Autodesk Fusion 360 part; units mm, degrees
(part 3 of 9)
sketch "Sketch5" plane through (0, 5.1, 0) normal (0, 1, 0) x (-1, 0, 0)
  line L0 (-250.175, 15.525) -> (-250.175, 3.525)
  arc A0 (-251.175, 2.525) -> (-250.175, 3.525) centre (-251.175, 3.525) ccw
  line L1 (-251.175, 2.525) -> (-263.175, 2.525)
  arc A1 (-264.175, 3.525) -> (-263.175, 2.525) centre (-263.175, 3.525) ccw
  line L2 (-264.175, 3.525) -> (-264.175, 15.525)
  arc A2 (-263.175, 16.525) -> (-264.175, 15.525) centre (-263.175, 15.525) ccw
  line L3 (-263.175, 16.525) -> (-251.175, 16.525)
  arc A3 (-250.175, 15.525) -> (-251.175, 16.525) centre (-251.175, 15.525) ccw
  line L4 (-216.8375, 53.625) -> (-216.8375, 41.625)
  arc A4 (-217.8375, 40.625) -> (-216.8375, 41.625) centre (-217.8375, 41.625) ccw
  line L5 (-217.8375, 40.625) -> (-229.8375, 40.625)
  arc A5 (-230.8375, 41.625) -> (-229.8375, 40.625) centre (-229.8375, 41.625) ccw
  line L6 (-230.8375, 41.625) -> (-230.8375, 53.625)
  arc A6 (-229.8375, 54.625) -> (-230.8375, 53.625) centre (-229.8375, 53.625) ccw
  line L7 (-229.8375, 54.625) -> (-217.8375, 54.625)
  arc A7 (-216.8375, 53.625) -> (-217.8375, 54.625) centre (-217.8375, 53.625) ccw
  line L8 (-188.2625, 34.575) -> (-188.2625, 22.575)
  arc A8 (-189.2625, 21.575) -> (-188.2625, 22.575) centre (-189.2625, 22.575) ccw
  line L9 (-189.2625, 21.575) -> (-201.2625, 21.575)
  arc A9 (-202.2625, 22.575) -> (-201.2625, 21.575) centre (-201.2625, 22.575) ccw
  line L10 (-202.2625, 22.575) -> (-202.2625, 34.575)
  arc A10 (-201.2625, 35.575) -> (-202.2625, 34.575) centre (-201.2625, 34.575) ccw
  line L11 (-201.2625, 35.575) -> (-189.2625, 35.575)
  arc A11 (-188.2625, 34.575) -> (-189.2625, 35.575) centre (-189.2625, 34.575) ccw
  line L12 (-178.7375, 53.625) -> (-178.7375, 41.625)
  arc A12 (-179.7375, 40.625) -> (-178.7375, 41.625) centre (-179.7375, 41.625) ccw
  line L13 (-179.7375, 40.625) -> (-191.7375, 40.625)
  arc A13 (-192.7375, 41.625) -> (-191.7375, 40.625) centre (-191.7375, 41.625) ccw
  line L14 (-192.7375, 41.625) -> (-192.7375, 53.625)
  arc A14 (-191.7375, 54.625) -> (-192.7375, 53.625) centre (-191.7375, 53.625) ccw
  line L15 (-191.7375, 54.625) -> (-179.7375, 54.625)
  arc A15 (-178.7375, 53.625) -> (-179.7375, 54.625) centre (-179.7375, 53.625) ccw
  line L16 (-140.6375, 53.625) -> (-140.6375, 41.625)
  arc A16 (-141.6375, 40.625) -> (-140.6375, 41.625) centre (-141.6375, 41.625) ccw
  line L17 (-141.6375, 40.625) -> (-153.6375, 40.625)
  arc A17 (-154.6375, 41.625) -> (-153.6375, 40.625) centre (-153.6375, 41.625) ccw
  line L18 (-154.6375, 41.625) -> (-154.6375, 53.625)
  arc A18 (-153.6375, 54.625) -> (-154.6375, 53.625) centre (-153.6375, 53.625) ccw
  line L19 (-153.6375, 54.625) -> (-141.6375, 54.625)
  arc A19 (-140.6375, 53.625) -> (-141.6375, 54.625) centre (-141.6375, 53.625) ccw
  line L20 (-131.1125, 34.575) -> (-131.1125, 22.575)
  arc A20 (-132.1125, 21.575) -> (-131.1125, 22.575) centre (-132.1125, 22.575) ccw
  line L21 (-132.1125, 21.575) -> (-144.1125, 21.575)
  arc A21 (-145.1125, 22.575) -> (-144.1125, 21.575) centre (-144.1125, 22.575) ccw
  line L22 (-145.1125, 22.575) -> (-145.1125, 34.575)
  arc A22 (-144.1125, 35.575) -> (-145.1125, 34.575) centre (-144.1125, 34.575) ccw
  line L23 (-144.1125, 35.575) -> (-132.1125, 35.575)
  arc A23 (-131.1125, 34.575) -> (-132.1125, 35.575) centre (-132.1125, 34.575) ccw
  line L24 (-107.3, 15.525) -> (-107.3, 3.525)
  arc A24 (-108.3, 2.525) -> (-107.3, 3.525) centre (-108.3, 3.525) ccw
  line L25 (-108.3, 2.525) -> (-120.3, 2.525)
  arc A25 (-121.3, 3.525) -> (-120.3, 2.525) centre (-120.3, 3.525) ccw
  line L26 (-121.3, 3.525) -> (-121.3, 15.525)
  arc A26 (-120.3, 16.525) -> (-121.3, 15.525) centre (-120.3, 15.525) ccw
  line L27 (-120.3, 16.525) -> (-108.3, 16.525)
  arc A27 (-107.3, 15.525) -> (-108.3, 16.525) centre (-108.3, 15.525) ccw
  line L28 (-122.2563, 73.675) -> (-92.0563, 73.675)
  arc A28 (-91.0563, 72.675) -> (-92.0563, 73.675) centre (-92.0563, 72.675) ccw
  line L29 (-91.0563, 72.675) -> (-91.0563, 60.675)
  arc A29 (-92.0563, 59.675) -> (-91.0563, 60.675) centre (-92.0563, 60.675) ccw
  line L30 (-92.0563, 59.675) -> (-122.2563, 59.675)
  arc A30 (-123.2563, 60.675) -> (-122.2563, 59.675) centre (-122.2563, 60.675) ccw
  line L31 (-123.2563, 60.675) -> (-123.2563, 72.675)
  arc A31 (-122.2563, 73.675) -> (-123.2563, 72.675) centre (-122.2563, 72.675) ccw
  line L32 (-69.2, 15.525) -> (-69.2, 3.525)
  arc A32 (-70.2, 2.525) -> (-69.2, 3.525) centre (-70.2, 3.525) ccw
  line L33 (-70.2, 2.525) -> (-82.2, 2.525)
  arc A33 (-83.2, 3.525) -> (-82.2, 2.525) centre (-82.2, 3.525) ccw
  line L34 (-83.2, 3.525) -> (-83.2, 15.525)
  arc A34 (-82.2, 16.525) -> (-83.2, 15.525) centre (-82.2, 15.525) ccw
  line L35 (-82.2, 16.525) -> (-70.2, 16.525)
  arc A35 (-69.2, 15.525) -> (-70.2, 16.525) centre (-70.2, 15.525) ccw
  line L36 (-45.3875, 53.625) -> (-45.3875, 41.625)
  arc A36 (-46.3875, 40.625) -> (-45.3875, 41.625) centre (-46.3875, 41.625) ccw
  line L37 (-46.3875, 40.625) -> (-58.3875, 40.625)
  arc A37 (-59.3875, 41.625) -> (-58.3875, 40.625) centre (-58.3875, 41.625) ccw
  line L38 (-59.3875, 41.625) -> (-59.3875, 53.625)
  arc A38 (-58.3875, 54.625) -> (-59.3875, 53.625) centre (-58.3875, 53.625) ccw
  line L39 (-58.3875, 54.625) -> (-46.3875, 54.625)
  arc A39 (-45.3875, 53.625) -> (-46.3875, 54.625) centre (-46.3875, 53.625) ccw
  line L40 (-9.6688, 34.575) -> (-9.6687, 22.575)
  arc A40 (-10.6687, 21.575) -> (-9.6687, 22.575) centre (-10.6688, 22.575) ccw
  line L41 (-10.6687, 21.575) -> (-22.6688, 21.575)
  arc A41 (-23.6688, 22.575) -> (-22.6688, 21.575) centre (-22.6687, 22.575) ccw
  line L42 (-23.6688, 22.575) -> (-23.6687, 34.575)
  arc A42 (-22.6687, 35.575) -> (-23.6687, 34.575) centre (-22.6687, 34.575) ccw
  line L43 (-22.6688, 35.575) -> (-10.6688, 35.575)
  arc A43 (-9.6688, 34.575) -> (-10.6687, 35.575) centre (-10.6688, 34.575) ccw
  line L44 (-44.1, 16.525) -> (-32.1, 16.525)
  arc A44 (-31.1, 15.525) -> (-32.1, 16.525) centre (-32.1, 15.525) ccw
  line L45 (-31.1, 15.525) -> (-31.1, 3.525)
  arc A45 (-32.1, 2.525) -> (-31.1, 3.525) centre (-32.1, 3.525) ccw
  line L46 (-32.1, 2.525) -> (-44.1, 2.525)
  arc A46 (-45.1, 3.525) -> (-44.1, 2.525) centre (-44.1, 3.525) ccw
  line L47 (-45.1, 3.525) -> (-45.1, 15.525)
  arc A47 (-44.1, 16.525) -> (-45.1, 15.525) centre (-44.1, 15.525) ccw
  line L48 (-40.625, 72.675) -> (-40.625, 60.675)
  arc A48 (-41.625, 59.675) -> (-40.625, 60.675) centre (-41.625, 60.675) ccw
  line L49 (-41.625, 59.675) -> (-53.625, 59.675)
  arc A49 (-54.625, 60.675) -> (-53.625, 59.675) centre (-53.625, 60.675) ccw
  line L50 (-54.625, 60.675) -> (-54.625, 72.675)
  arc A50 (-53.625, 73.675) -> (-54.625, 72.675) centre (-53.625, 72.675) ccw
  line L51 (-53.625, 73.675) -> (-41.625, 73.675)
  arc A51 (-40.625, 72.675) -> (-41.625, 73.675) centre (-41.625, 72.675) ccw
  line L52 (-54.9125, 34.575) -> (-54.9125, 22.575)
  arc A52 (-55.9125, 21.575) -> (-54.9125, 22.575) centre (-55.9125, 22.575) ccw
  line L53 (-55.9125, 21.575) -> (-67.9125, 21.575)
  arc A53 (-68.9125, 22.575) -> (-67.9125, 21.575) centre (-67.9125, 22.575) ccw
  line L54 (-68.9125, 22.575) -> (-68.9125, 34.575)
  arc A54 (-67.9125, 35.575) -> (-68.9125, 34.575) centre (-67.9125, 34.575) ccw
  line L55 (-67.9125, 35.575) -> (-55.9125, 35.575)
  arc A55 (-54.9125, 34.575) -> (-55.9125, 35.575) centre (-55.9125, 34.575) ccw
  line L56 (-66.8188, 72.675) -> (-66.8188, 60.675)
  arc A56 (-67.8188, 59.675) -> (-66.8188, 60.675) centre (-67.8188, 60.675) ccw
  line L57 (-67.8188, 59.675) -> (-79.8188, 59.675)
  arc A57 (-80.8188, 60.675) -> (-79.8188, 59.675) centre (-79.8188, 60.675) ccw
  line L58 (-80.8187, 60.675) -> (-80.8187, 72.675)
  arc A58 (-79.8188, 73.675) -> (-80.8188, 72.675) centre (-79.8188, 72.675) ccw
  line L59 (-79.8188, 73.675) -> (-67.8188, 73.675)
  arc A59 (-66.8188, 72.675) -> (-67.8188, 73.675) centre (-67.8188, 72.675) ccw
  line L60 (-88.25, 15.525) -> (-88.25, 3.525)
  arc A60 (-89.25, 2.525) -> (-88.25, 3.525) centre (-89.25, 3.525) ccw
  line L61 (-89.25, 2.525) -> (-101.25, 2.525)
  arc A61 (-102.25, 3.525) -> (-101.25, 2.525) centre (-101.25, 3.525) ccw
  line L62 (-102.25, 3.525) -> (-102.25, 15.525)
  arc A62 (-101.25, 16.525) -> (-102.25, 15.525) centre (-101.25, 15.525) ccw
  line L63 (-101.25, 16.525) -> (-89.25, 16.525)
  arc A63 (-88.25, 15.525) -> (-89.25, 16.525) centre (-89.25, 15.525) ccw
  line L64 (-121.5875, 53.625) -> (-121.5875, 41.625)
  arc A64 (-122.5875, 40.625) -> (-121.5875, 41.625) centre (-122.5875, 41.625) ccw
  line L65 (-122.5875, 40.625) -> (-134.5875, 40.625)
  arc A65 (-135.5875, 41.625) -> (-134.5875, 40.625) centre (-134.5875, 41.625) ccw
  line L66 (-135.5875, 41.625) -> (-135.5875, 53.625)
  arc A66 (-134.5875, 54.625) -> (-135.5875, 53.625) centre (-134.5875, 53.625) ccw
  line L67 (-134.5875, 54.625) -> (-122.5875, 54.625)
  arc A67 (-121.5875, 53.625) -> (-122.5875, 54.625) centre (-122.5875, 53.625) ccw
  line L68 (-150.1625, 34.575) -> (-150.1625, 22.575)
  arc A68 (-151.1625, 21.575) -> (-150.1625, 22.575) centre (-151.1625, 22.575) ccw
  line L69 (-151.1625, 21.575) -> (-163.1625, 21.575)
  arc A69 (-164.1625, 22.575) -> (-163.1625, 21.575) centre (-163.1625, 22.575) ccw
  line L70 (-164.1625, 22.575) -> (-164.1625, 34.575)
  arc A70 (-163.1625, 35.575) -> (-164.1625, 34.575) centre (-163.1625, 34.575) ccw
  line L71 (-163.1625, 35.575) -> (-151.1625, 35.575)
  arc A71 (-150.1625, 34.575) -> (-151.1625, 35.575) centre (-151.1625, 34.575) ccw
  line L72 (-171.5938, 72.675) -> (-171.5937, 60.675)
  arc A72 (-172.5937, 59.675) -> (-171.5937, 60.675) centre (-172.5937, 60.675) ccw
  line L73 (-172.5938, 59.675) -> (-184.5938, 59.675)
  arc A73 (-185.5938, 60.675) -> (-184.5938, 59.675) centre (-184.5938, 60.675) ccw
  line L74 (-185.5938, 60.675) -> (-185.5937, 72.675)
  arc A74 (-184.5938, 73.675) -> (-185.5937, 72.675) centre (-184.5937, 72.675) ccw
  line L75 (-184.5938, 73.675) -> (-172.5937, 73.675)
  arc A75 (-171.5938, 72.675) -> (-172.5937, 73.675) centre (-172.5937, 72.675) ccw
  line L76 (-183.5, 15.525) -> (-183.5, 3.525)
  arc A76 (-184.5, 2.525) -> (-183.5, 3.525) centre (-184.5, 3.525) ccw
  line L77 (-184.5, 2.525) -> (-196.5, 2.525)
  arc A77 (-197.5, 3.525) -> (-196.5, 2.525) centre (-196.5, 3.525) ccw
  line L78 (-197.5, 3.525) -> (-197.5, 15.525)
  arc A78 (-196.5, 16.525) -> (-197.5, 15.525) centre (-196.5, 15.525) ccw
  line L79 (-196.5, 16.525) -> (-184.5, 16.525)
  arc A79 (-183.5, 15.525) -> (-184.5, 16.525) centre (-184.5, 15.525) ccw
  line L80 (-223.9813, 72.675) -> (-223.9813, 60.675)
  arc A80 (-224.9813, 59.675) -> (-223.9812, 60.675) centre (-224.9812, 60.675) ccw
  line L81 (-224.9813, 59.675) -> (-236.9813, 59.675)
  arc A81 (-237.9813, 60.675) -> (-236.9813, 59.675) centre (-236.9813, 60.675) ccw
  line L82 (-237.9813, 60.675) -> (-237.9812, 72.675)
  arc A82 (-236.9813, 73.675) -> (-237.9813, 72.675) centre (-236.9813, 72.675) ccw
  line L83 (-236.9813, 73.675) -> (-224.9813, 73.675)
  arc A83 (-223.9813, 72.675) -> (-224.9813, 73.675) centre (-224.9812, 72.675) ccw
  line L84 (-226.3625, 15.525) -> (-226.3625, 3.525)
  arc A84 (-227.3625, 2.525) -> (-226.3625, 3.525) centre (-227.3625, 3.525) ccw
  line L85 (-227.3625, 2.525) -> (-239.3625, 2.525)
  arc A85 (-240.3625, 3.525) -> (-239.3625, 2.525) centre (-239.3625, 3.525) ccw
  line L86 (-240.3625, 3.525) -> (-240.3625, 15.525)
  arc A86 (-239.3625, 16.525) -> (-240.3625, 15.525) centre (-239.3625, 15.525) ccw
  line L87 (-239.3625, 16.525) -> (-227.3625, 16.525)
  arc A87 (-226.3625, 15.525) -> (-227.3625, 16.525) centre (-227.3625, 15.525) ccw
  line L88 (-260.3688, 35.575) -> (-230.1688, 35.575)
  arc A88 (-229.1688, 34.575) -> (-230.1688, 35.575) centre (-230.1688, 34.575) ccw
  line L89 (-229.1688, 34.575) -> (-229.1688, 22.575)
  arc A89 (-230.1688, 21.575) -> (-229.1688, 22.575) centre (-230.1688, 22.575) ccw
  line L90 (-230.1688, 21.575) -> (-260.3688, 21.575)
  arc A90 (-261.3688, 22.575) -> (-260.3688, 21.575) centre (-260.3688, 22.575) ccw
  line L91 (-261.3688, 22.575) -> (-261.3688, 34.575)
  arc A91 (-260.3688, 35.575) -> (-261.3688, 34.575) centre (-260.3687, 34.575) ccw
  line L92 (-207.3125, 34.575) -> (-207.3125, 22.575)
  arc A92 (-208.3125, 21.575) -> (-207.3125, 22.575) centre (-208.3125, 22.575) ccw
  line L93 (-208.3125, 21.575) -> (-220.3125, 21.575)
  arc A93 (-221.3125, 22.575) -> (-220.3125, 21.575) centre (-220.3125, 22.575) ccw
  line L94 (-221.3125, 22.575) -> (-221.3125, 34.575)
  arc A94 (-220.3125, 35.575) -> (-221.3125, 34.575) centre (-220.3125, 34.575) ccw
  line L95 (-220.3125, 35.575) -> (-208.3125, 35.575)
  arc A95 (-207.3125, 34.575) -> (-208.3125, 35.575) centre (-208.3125, 34.575) ccw
  line L96 (-197.7875, 53.625) -> (-197.7875, 41.625)
  arc A96 (-198.7875, 40.625) -> (-197.7875, 41.625) centre (-198.7875, 41.625) ccw
  line L97 (-198.7875, 40.625) -> (-210.7875, 40.625)
  arc A97 (-211.7875, 41.625) -> (-210.7875, 40.625) centre (-210.7875, 41.625) ccw
  line L98 (-211.7875, 41.625) -> (-211.7875, 53.625)
  arc A98 (-210.7875, 54.625) -> (-211.7875, 53.625) centre (-210.7875, 53.625) ccw
  line L99 (-210.7875, 54.625) -> (-198.7875, 54.625)
  arc A99 (-197.7875, 53.625) -> (-198.7875, 54.625) centre (-198.7875, 53.625) ccw
  line L100 (-169.2125, 34.575) -> (-169.2125, 22.575)
  arc A100 (-170.2125, 21.575) -> (-169.2125, 22.575) centre (-170.2125, 22.575) ccw
  line L101 (-170.2125, 21.575) -> (-182.2125, 21.575)
  arc A101 (-183.2125, 22.575) -> (-182.2125, 21.575) centre (-182.2125, 22.575) ccw
  line L102 (-183.2125, 22.575) -> (-183.2125, 34.575)
  arc A102 (-182.2125, 35.575) -> (-183.2125, 34.575) centre (-182.2125, 34.575) ccw
  line L103 (-182.2125, 35.575) -> (-170.2125, 35.575)
  arc A103 (-169.2125, 34.575) -> (-170.2125, 35.575) centre (-170.2125, 34.575) ccw
  line L104 (-132.5375, 59.675) -> (-162.7375, 59.675)
  arc A104 (-163.7375, 60.675) -> (-162.7375, 59.675) centre (-162.7375, 60.675) ccw
  line L105 (-163.7375, 60.675) -> (-163.7375, 72.675)
  arc A105 (-162.7375, 73.675) -> (-163.7375, 72.675) centre (-162.7375, 72.675) ccw
  line L106 (-162.7375, 73.675) -> (-132.5375, 73.675)
  arc A106 (-131.5375, 72.675) -> (-132.5375, 73.675) centre (-132.5375, 72.675) ccw
  line L107 (-131.5375, 72.675) -> (-131.5375, 60.675)
  arc A107 (-132.5375, 59.675) -> (-131.5375, 60.675) centre (-132.5375, 60.675) ccw
  line L108 (-126.35, 15.525) -> (-126.35, 3.525)
  arc A108 (-127.35, 2.525) -> (-126.35, 3.525) centre (-127.35, 3.525) ccw
  line L109 (-127.35, 2.525) -> (-139.35, 2.525)
  arc A109 (-140.35, 3.525) -> (-139.35, 2.525) centre (-139.35, 3.525) ccw
  line L110 (-140.35, 3.525) -> (-140.35, 15.525)
  arc A110 (-139.35, 16.525) -> (-140.35, 15.525) centre (-139.35, 15.525) ccw
  line L111 (-139.35, 16.525) -> (-127.35, 16.525)
  arc A111 (-126.35, 15.525) -> (-127.35, 16.525) centre (-127.35, 15.525) ccw
  line L112 (-112.0625, 34.575) -> (-112.0625, 22.575)
  arc A112 (-113.0625, 21.575) -> (-112.0625, 22.575) centre (-113.0625, 22.575) ccw
  line L113 (-113.0625, 21.575) -> (-125.0625, 21.575)
  arc A113 (-126.0625, 22.575) -> (-125.0625, 21.575) centre (-125.0625, 22.575) ccw
  line L114 (-126.0625, 22.575) -> (-126.0625, 34.575)
  arc A114 (-125.0625, 35.575) -> (-126.0625, 34.575) centre (-125.0625, 34.575) ccw
  line L115 (-125.0625, 35.575) -> (-113.0625, 35.575)
  arc A115 (-112.0625, 34.575) -> (-113.0625, 35.575) centre (-113.0625, 34.575) ccw
  line L116 (-83.4875, 53.625) -> (-83.4875, 41.625)
  arc A116 (-84.4875, 40.625) -> (-83.4875, 41.625) centre (-84.4875, 41.625) ccw
  line L117 (-84.4875, 40.625) -> (-96.4875, 40.625)
  arc A117 (-97.4875, 41.625) -> (-96.4875, 40.625) centre (-96.4875, 41.625) ccw
  line L118 (-97.4875, 41.625) -> (-97.4875, 53.625)
  arc A118 (-96.4875, 54.625) -> (-97.4875, 53.625) centre (-96.4875, 53.625) ccw
  line L119 (-96.4875, 54.625) -> (-84.4875, 54.625)
  arc A119 (-83.4875, 53.625) -> (-84.4875, 54.625) centre (-84.4875, 53.625) ccw
  line L120 (-73.9625, 34.575) -> (-73.9625, 22.575)
  arc A120 (-74.9625, 21.575) -> (-73.9625, 22.575) centre (-74.9625, 22.575) ccw
  line L121 (-74.9625, 21.575) -> (-86.9625, 21.575)
  arc A121 (-87.9625, 22.575) -> (-86.9625, 21.575) centre (-86.9625, 22.575) ccw
  line L122 (-87.9625, 22.575) -> (-87.9625, 34.575)
  arc A122 (-86.9625, 35.575) -> (-87.9625, 34.575) centre (-86.9625, 34.575) ccw
  line L123 (-86.9625, 35.575) -> (-74.9625, 35.575)
  arc A123 (-73.9625, 34.575) -> (-74.9625, 35.575) centre (-74.9625, 34.575) ccw
  line L124 (-35.8625, 34.575) -> (-35.8625, 22.575)
  arc A124 (-36.8625, 21.575) -> (-35.8625, 22.575) centre (-36.8625, 22.575) ccw
  line L125 (-36.8625, 21.575) -> (-48.8625, 21.575)
  arc A125 (-49.8625, 22.575) -> (-48.8625, 21.575) centre (-48.8625, 22.575) ccw
  line L126 (-49.8625, 22.575) -> (-49.8625, 34.575)
  arc A126 (-48.8625, 35.575) -> (-49.8625, 34.575) centre (-48.8625, 34.575) ccw
  line L127 (-48.8625, 35.575) -> (-36.8625, 35.575)
  arc A127 (-35.8625, 34.575) -> (-36.8625, 35.575) centre (-36.8625, 34.575) ccw
  line L128 (-6.3312, 40.625) -> (-36.5313, 40.625)
  arc A128 (-37.5313, 41.625) -> (-36.5313, 40.625) centre (-36.5313, 41.625) ccw
  line L129 (-37.5312, 41.625) -> (-37.5312, 53.625)
  arc A129 (-36.5313, 54.625) -> (-37.5313, 53.625) centre (-36.5313, 53.625) ccw
  line L130 (-36.5313, 54.625) -> (-6.3313, 54.625)
  arc A130 (-5.3313, 53.625) -> (-6.3313, 54.625) centre (-6.3312, 53.625) ccw
  line L131 (-5.3313, 53.625) -> (-5.3312, 41.625)
  arc A131 (-6.3312, 40.625) -> (-5.3312, 41.625) centre (-6.3312, 41.625) ccw
  line L132 (-7.2875, 15.525) -> (-7.2875, 3.525)
  arc A132 (-8.2875, 2.525) -> (-7.2875, 3.525) centre (-8.2875, 3.525) ccw
  line L133 (-8.2875, 2.525) -> (-20.2875, 2.525)
  arc A133 (-21.2875, 3.525) -> (-20.2875, 2.525) centre (-20.2875, 3.525) ccw
  line L134 (-21.2875, 3.525) -> (-21.2875, 15.525)
  arc A134 (-20.2875, 16.525) -> (-21.2875, 15.525) centre (-20.2875, 15.525) ccw
  line L135 (-20.2875, 16.525) -> (-8.2875, 16.525)
  arc A135 (-7.2875, 15.525) -> (-8.2875, 16.525) centre (-8.2875, 15.525) ccw
  line L136 (-14.4313, 72.675) -> (-14.4313, 60.675)
  arc A136 (-15.4313, 59.675) -> (-14.4313, 60.675) centre (-15.4312, 60.675) ccw
  line L137 (-15.4313, 59.675) -> (-27.4313, 59.675)
  arc A137 (-28.4313, 60.675) -> (-27.4313, 59.675) centre (-27.4313, 60.675) ccw
  line L138 (-28.4313, 60.675) -> (-28.4312, 72.675)
  arc A138 (-27.4313, 73.675) -> (-28.4312, 72.675) centre (-27.4312, 72.675) ccw
  line L139 (-27.4313, 73.675) -> (-15.4313, 73.675)
  arc A139 (-14.4313, 72.675) -> (-15.4313, 73.675) centre (-15.4313, 72.675) ccw
  line L140 (-50.15, 15.525) -> (-50.15, 3.525)
  arc A140 (-51.15, 2.525) -> (-50.15, 3.525) centre (-51.15, 3.525) ccw
  line L141 (-51.15, 2.525) -> (-63.15, 2.525)
  arc A141 (-64.15, 3.525) -> (-63.15, 2.525) centre (-63.15, 3.525) ccw
  line L142 (-64.15, 3.525) -> (-64.15, 15.525)
  arc A142 (-63.15, 16.525) -> (-64.15, 15.525) centre (-63.15, 15.525) ccw
  line L143 (-63.15, 16.525) -> (-51.15, 16.525)
  arc A143 (-50.15, 15.525) -> (-51.15, 16.525) centre (-51.15, 15.525) ccw
  line L144 (-64.4375, 53.625) -> (-64.4375, 41.625)
  arc A144 (-65.4375, 40.625) -> (-64.4375, 41.625) centre (-65.4375, 41.625) ccw
  line L145 (-65.4375, 40.625) -> (-77.4375, 40.625)
  arc A145 (-78.4375, 41.625) -> (-77.4375, 40.625) centre (-77.4375, 41.625) ccw
  line L146 (-78.4375, 41.625) -> (-78.4375, 53.625)
  arc A146 (-77.4375, 54.625) -> (-78.4375, 53.625) centre (-77.4375, 53.625) ccw
  line L147 (-77.4375, 54.625) -> (-65.4375, 54.625)
  arc A147 (-64.4375, 53.625) -> (-65.4375, 54.625) centre (-65.4375, 53.625) ccw
  line L148 (-93.0125, 34.575) -> (-93.0125, 22.575)
  arc A148 (-94.0125, 21.575) -> (-93.0125, 22.575) centre (-94.0125, 22.575) ccw
  line L149 (-94.0125, 21.575) -> (-106.0125, 21.575)
  arc A149 (-107.0125, 22.575) -> (-106.0125, 21.575) centre (-106.0125, 22.575) ccw
  line L150 (-107.0125, 22.575) -> (-107.0125, 34.575)
  arc A150 (-106.0125, 35.575) -> (-107.0125, 34.575) centre (-106.0125, 34.575) ccw
  line L151 (-106.0125, 35.575) -> (-94.0125, 35.575)
  arc A151 (-93.0125, 34.575) -> (-94.0125, 35.575) centre (-94.0125, 34.575) ccw
  line L152 (-102.5375, 53.625) -> (-102.5375, 41.625)
  arc A152 (-103.5375, 40.625) -> (-102.5375, 41.625) centre (-103.5375, 41.625) ccw
  line L153 (-103.5375, 40.625) -> (-115.5375, 40.625)
  arc A153 (-116.5375, 41.625) -> (-115.5375, 40.625) centre (-115.5375, 41.625) ccw
  line L154 (-116.5375, 41.625) -> (-116.5375, 53.625)
  arc A154 (-115.5375, 54.625) -> (-116.5375, 53.625) centre (-115.5375, 53.625) ccw
  line L155 (-115.5375, 54.625) -> (-103.5375, 54.625)
  arc A155 (-102.5375, 53.625) -> (-103.5375, 54.625) centre (-103.5375, 53.625) ccw
  line L156 (-145.4, 15.525) -> (-145.4, 3.525)
  arc A156 (-146.4, 2.525) -> (-145.4, 3.525) centre (-146.4, 3.525) ccw
  line L157 (-146.4, 2.525) -> (-158.4, 2.525)
  arc A157 (-159.4, 3.525) -> (-158.4, 2.525) centre (-158.4, 3.525) ccw
  line L158 (-159.4, 3.525) -> (-159.4, 15.525)
  arc A158 (-158.4, 16.525) -> (-159.4, 15.525) centre (-158.4, 15.525) ccw
  line L159 (-158.4, 16.525) -> (-146.4, 16.525)
  arc A159 (-145.4, 15.525) -> (-146.4, 16.525) centre (-146.4, 15.525) ccw
  line L160 (-159.6875, 53.625) -> (-159.6875, 41.625)
  arc A160 (-160.6875, 40.625) -> (-159.6875, 41.625) centre (-160.6875, 41.625) ccw
  line L161 (-160.6875, 40.625) -> (-172.6875, 40.625)
  arc A161 (-173.6875, 41.625) -> (-172.6875, 40.625) centre (-172.6875, 41.625) ccw
  line L162 (-173.6875, 41.625) -> (-173.6875, 53.625)
  arc A162 (-172.6875, 54.625) -> (-173.6875, 53.625) centre (-172.6875, 53.625) ccw
  line L163 (-172.6875, 54.625) -> (-160.6875, 54.625)
  arc A163 (-159.6875, 53.625) -> (-160.6875, 54.625) centre (-160.6875, 53.625) ccw
  line L164 (-164.45, 15.525) -> (-164.45, 3.525)
  arc A164 (-165.45, 2.525) -> (-164.45, 3.525) centre (-165.45, 3.525) ccw
  line L165 (-165.45, 2.525) -> (-177.45, 2.525)
  arc A165 (-178.45, 3.525) -> (-177.45, 2.525) centre (-177.45, 3.525) ccw
  line L166 (-178.45, 3.525) -> (-178.45, 15.525)
  arc A166 (-177.45, 16.525) -> (-178.45, 15.525) centre (-177.45, 15.525) ccw
  line L167 (-177.45, 16.525) -> (-165.45, 16.525)
  arc A167 (-164.45, 15.525) -> (-165.45, 16.525) centre (-165.45, 15.525) ccw
  line L168 (-197.7875, 72.675) -> (-197.7875, 60.675)
  arc A168 (-198.7875, 59.675) -> (-197.7875, 60.675) centre (-198.7875, 60.675) ccw
  line L169 (-198.7875, 59.675) -> (-210.7875, 59.675)
  arc A169 (-211.7875, 60.675) -> (-210.7875, 59.675) centre (-210.7875, 60.675) ccw
  line L170 (-211.7875, 60.675) -> (-211.7875, 72.675)
  arc A170 (-210.7875, 73.675) -> (-211.7875, 72.675) centre (-210.7875, 72.675) ccw
  line L171 (-210.7875, 73.675) -> (-198.7875, 73.675)
  arc A171 (-197.7875, 72.675) -> (-198.7875, 73.675) centre (-198.7875, 72.675) ccw
  line L172 (-202.55, 15.525) -> (-202.55, 3.525)
  arc A172 (-203.55, 2.525) -> (-202.55, 3.525) centre (-203.55, 3.525) ccw
  line L173 (-203.55, 2.525) -> (-215.55, 2.525)
  arc A173 (-216.55, 3.525) -> (-215.55, 2.525) centre (-215.55, 3.525) ccw
  line L174 (-216.55, 3.525) -> (-216.55, 15.525)
  arc A174 (-215.55, 16.525) -> (-216.55, 15.525) centre (-215.55, 15.525) ccw
  line L175 (-215.55, 16.525) -> (-203.55, 16.525)
  arc A175 (-202.55, 15.525) -> (-203.55, 16.525) centre (-203.55, 15.525) ccw
  line L176 (-243.0312, 53.625) -> (-243.0312, 41.625)
  arc A176 (-244.0312, 40.625) -> (-243.0313, 41.625) centre (-244.0313, 41.625) ccw
  line L177 (-244.0312, 40.625) -> (-256.0312, 40.625)
  arc A177 (-257.0312, 41.625) -> (-256.0312, 40.625) centre (-256.0312, 41.625) ccw
  line L178 (-257.0312, 41.625) -> (-257.0312, 53.625)
  arc A178 (-256.0312, 54.625) -> (-257.0312, 53.625) centre (-256.0312, 53.625) ccw
  line L179 (-256.0312, 54.625) -> (-244.0312, 54.625)
  arc A179 (-243.0313, 53.625) -> (-244.0312, 54.625) centre (-244.0312, 53.625) ccw
  arc A180 (-263.7, 57.15) -> (-266.7, 54.15) centre (-263.7, 54.15) ccw
  line L180 (-266.7, 54.15) -> (-266.7, 3)
  arc A181 (-266.7, 3) -> (-263.7, 0) centre (-263.7, 3) ccw
  line L181 (-263.7, 0) -> (-3, 0)
  arc A182 (-3, 0) -> (0, 3) centre (-3, 3) ccw
  line L182 (0, 3) -> (0, 54.15)
  arc A183 (0, 54.15) -> (-3, 57.15) centre (-3, 54.15) ccw
  line L183 (-3, 57.15) -> (-8.525, 57.15)
  arc A184 (-9.525, 58.15) -> (-8.525, 57.15) centre (-8.525, 58.15) ccw
  line L184 (-9.525, 58.15) -> (-9.525, 73.2)
  arc A185 (-9.525, 73.2) -> (-12.525, 76.2) centre (-12.525, 73.2) ccw
  line L185 (-12.525, 76.2) -> (-239.8875, 76.2)
  arc A186 (-239.8875, 76.2) -> (-242.8875, 73.2) centre (-239.8875, 73.2) ccw
  line L186 (-242.8875, 73.2) -> (-242.8875, 58.15)
  arc A187 (-243.8875, 57.15) -> (-242.8875, 58.15) centre (-243.8875, 58.15) ccw
  line L187 (-243.8875, 57.15) -> (-263.7, 57.15)
  circle A188 centre (-47.625, 9.525) radius 2.5
  circle A189 centre (-245.269, 9.525) radius 2.5
  circle A190 centre (-128.588, 37.025) radius 2.5
  circle A191 centre (-32.525, 66.675) radius 2.5
  circle A192 centre (-220.025, 66.675) radius 2.5
  point P0 (-9.525, 9.525)
  dimension "d82" = 9.525
  dimension "d83" = 9.525
  dimension "d84" = 5
  dimension "d85" = 38.1
  dimension "d86" = 5
  dimension "d87" = 235.744
  dimension "d88" = 5
  dimension "d89" = 119.063
  dimension "d90" = 27.5
  dimension "d91" = 5
  dimension "d92" = 5
  dimension "d93" = 57.15
  dimension "d94" = 57.15
  dimension "d95" = 23
  dimension "d96" = 210.5
  measures "d82" distance of L181 P0
  measures "d83" distance of L182 P0
  measures "d84" diameter of A188
  measures "d85" distance of P0 A188.centre
  measures "d86" diameter of A189
  measures "d87" distance of P0 A189.centre
  measures "d88" diameter of A190
  measures "d89" horizontal distance of P0 A190.centre
  measures "d90" vertical distance of P0 A190.centre
  measures "d91" diameter of A191
  measures "d92" diameter of A192
  measures "d93" vertical distance of P0 A191.centre
  measures "d94" vertical distance of P0 A192.centre
  measures "d95" horizontal distance of P0 A191.centre
  measures "d96" horizontal distance of P0 A192.centre
hole "Hole1" at (245.269, 5.1, 9.525) at (220.025, 5.1, 66.675) at (128.588, 5.1, 37.025) at (47.625, 5.1, 9.525) at (32.525, 5.1, 66.675) direction (0, -1, 0) diameter 2.5 depth 5.1 tip angle 118 counterbore diameter 5 counterbore depth 1.5
sketch "Sketch6" plane through (0, 5.1, 0) normal (0, 1, 0) x (-1, 0, 0)
  circle A0 centre (-47.625, 9.525) radius 2.5
  circle A1 centre (-220.025, 66.675) radius 2.5
  circle A2 centre (-245.269, 9.525) radius 2.5
  circle A3 centre (-128.588, 37.025) radius 2.5
  circle A4 centre (-32.525, 66.675) radius 2.5
  line L0 (-250.175, 15.525) -> (-250.175, 3.525)
  arc A5 (-251.175, 2.525) -> (-250.175, 3.525) centre (-251.175, 3.525) ccw
  line L1 (-251.175, 2.525) -> (-263.175, 2.525)
  arc A6 (-264.175, 3.525) -> (-263.175, 2.525) centre (-263.175, 3.525) ccw
  line L2 (-264.175, 3.525) -> (-264.175, 15.525)
  arc A7 (-263.175, 16.525) -> (-264.175, 15.525) centre (-263.175, 15.525) ccw
  line L3 (-263.175, 16.525) -> (-251.175, 16.525)
  arc A8 (-250.175, 15.525) -> (-251.175, 16.525) centre (-251.175, 15.525) ccw
  line L4 (-216.8375, 53.625) -> (-216.8375, 41.625)
  arc A9 (-217.8375, 40.625) -> (-216.8375, 41.625) centre (-217.8375, 41.625) ccw
  line L5 (-217.8375, 40.625) -> (-229.8375, 40.625)
  arc A10 (-230.8375, 41.625) -> (-229.8375, 40.625) centre (-229.8375, 41.625) ccw
  line L6 (-230.8375, 41.625) -> (-230.8375, 53.625)
  arc A11 (-229.8375, 54.625) -> (-230.8375, 53.625) centre (-229.8375, 53.625) ccw
  line L7 (-229.8375, 54.625) -> (-217.8375, 54.625)
  arc A12 (-216.8375, 53.625) -> (-217.8375, 54.625) centre (-217.8375, 53.625) ccw
  line L8 (-188.2625, 34.575) -> (-188.2625, 22.575)
  arc A13 (-189.2625, 21.575) -> (-188.2625, 22.575) centre (-189.2625, 22.575) ccw
  line L9 (-189.2625, 21.575) -> (-201.2625, 21.575)
  arc A14 (-202.2625, 22.575) -> (-201.2625, 21.575) centre (-201.2625, 22.575) ccw
  line L10 (-202.2625, 22.575) -> (-202.2625, 34.575)
  arc A15 (-201.2625, 35.575) -> (-202.2625, 34.575) centre (-201.2625, 34.575) ccw
  line L11 (-201.2625, 35.575) -> (-189.2625, 35.575)
  arc A16 (-188.2625, 34.575) -> (-189.2625, 35.575) centre (-189.2625, 34.575) ccw
  line L12 (-178.7375, 53.625) -> (-178.7375, 41.625)
  arc A17 (-179.7375, 40.625) -> (-178.7375, 41.625) centre (-179.7375, 41.625) ccw
  line L13 (-179.7375, 40.625) -> (-191.7375, 40.625)
  arc A18 (-192.7375, 41.625) -> (-191.7375, 40.625) centre (-191.7375, 41.625) ccw
  line L14 (-192.7375, 41.625) -> (-192.7375, 53.625)
  arc A19 (-191.7375, 54.625) -> (-192.7375, 53.625) centre (-191.7375, 53.625) ccw
  line L15 (-191.7375, 54.625) -> (-179.7375, 54.625)
  arc A20 (-178.7375, 53.625) -> (-179.7375, 54.625) centre (-179.7375, 53.625) ccw
  line L16 (-140.6375, 53.625) -> (-140.6375, 41.625)
  arc A21 (-141.6375, 40.625) -> (-140.6375, 41.625) centre (-141.6375, 41.625) ccw
  line L17 (-141.6375, 40.625) -> (-153.6375, 40.625)
  arc A22 (-154.6375, 41.625) -> (-153.6375, 40.625) centre (-153.6375, 41.625) ccw
  line L18 (-154.6375, 41.625) -> (-154.6375, 53.625)
  arc A23 (-153.6375, 54.625) -> (-154.6375, 53.625) centre (-153.6375, 53.625) ccw
  line L19 (-153.6375, 54.625) -> (-141.6375, 54.625)
  arc A24 (-140.6375, 53.625) -> (-141.6375, 54.625) centre (-141.6375, 53.625) ccw
  line L20 (-131.1125, 34.575) -> (-131.1125, 22.575)
  arc A25 (-132.1125, 21.575) -> (-131.1125, 22.575) centre (-132.1125, 22.575) ccw
  line L21 (-132.1125, 21.575) -> (-144.1125, 21.575)
  arc A26 (-145.1125, 22.575) -> (-144.1125, 21.575) centre (-144.1125, 22.575) ccw
  line L22 (-145.1125, 22.575) -> (-145.1125, 34.575)
  arc A27 (-144.1125, 35.575) -> (-145.1125, 34.575) centre (-144.1125, 34.575) ccw
  line L23 (-144.1125, 35.575) -> (-132.1125, 35.575)
  arc A28 (-131.1125, 34.575) -> (-132.1125, 35.575) centre (-132.1125, 34.575) ccw
  line L24 (-107.3, 15.525) -> (-107.3, 3.525)
  arc A29 (-108.3, 2.525) -> (-107.3, 3.525) centre (-108.3, 3.525) ccw
  line L25 (-108.3, 2.525) -> (-120.3, 2.525)
  arc A30 (-121.3, 3.525) -> (-120.3, 2.525) centre (-120.3, 3.525) ccw
  line L26 (-121.3, 3.525) -> (-121.3, 15.525)
  arc A31 (-120.3, 16.525) -> (-121.3, 15.525) centre (-120.3, 15.525) ccw
  line L27 (-120.3, 16.525) -> (-108.3, 16.525)
  arc A32 (-107.3, 15.525) -> (-108.3, 16.525) centre (-108.3, 15.525) ccw
  line L28 (-122.2563, 73.675) -> (-92.0563, 73.675)
  arc A33 (-91.0563, 72.675) -> (-92.0563, 73.675) centre (-92.0563, 72.675) ccw
  line L29 (-91.0563, 72.675) -> (-91.0563, 60.675)
  arc A34 (-92.0563, 59.675) -> (-91.0563, 60.675) centre (-92.0563, 60.675) ccw
  line L30 (-92.0563, 59.675) -> (-122.2563, 59.675)
  arc A35 (-123.2563, 60.675) -> (-122.2563, 59.675) centre (-122.2563, 60.675) ccw
  line L31 (-123.2563, 60.675) -> (-123.2563, 72.675)
  arc A36 (-122.2563, 73.675) -> (-123.2563, 72.675) centre (-122.2563, 72.675) ccw
  line L32 (-69.2, 15.525) -> (-69.2, 3.525)
  arc A37 (-70.2, 2.525) -> (-69.2, 3.525) centre (-70.2, 3.525) ccw
  line L33 (-70.2, 2.525) -> (-82.2, 2.525)
  arc A38 (-83.2, 3.525) -> (-82.2, 2.525) centre (-82.2, 3.525) ccw
  line L34 (-83.2, 3.525) -> (-83.2, 15.525)
  arc A39 (-82.2, 16.525) -> (-83.2, 15.525) centre (-82.2, 15.525) ccw
  line L35 (-82.2, 16.525) -> (-70.2, 16.525)
  arc A40 (-69.2, 15.525) -> (-70.2, 16.525) centre (-70.2, 15.525) ccw
  line L36 (-45.3875, 53.625) -> (-45.3875, 41.625)
  arc A41 (-46.3875, 40.625) -> (-45.3875, 41.625) centre (-46.3875, 41.625) ccw
  line L37 (-46.3875, 40.625) -> (-58.3875, 40.625)
  arc A42 (-59.3875, 41.625) -> (-58.3875, 40.625) centre (-58.3875, 41.625) ccw
  line L38 (-59.3875, 41.625) -> (-59.3875, 53.625)
  arc A43 (-58.3875, 54.625) -> (-59.3875, 53.625) centre (-58.3875, 53.625) ccw
  line L39 (-58.3875, 54.625) -> (-46.3875, 54.625)
  arc A44 (-45.3875, 53.625) -> (-46.3875, 54.625) centre (-46.3875, 53.625) ccw
  line L40 (-9.6688, 34.575) -> (-9.6687, 22.575)
  arc A45 (-10.6687, 21.575) -> (-9.6687, 22.575) centre (-10.6688, 22.575) ccw
  line L41 (-10.6687, 21.575) -> (-22.6688, 21.575)
  arc A46 (-23.6688, 22.575) -> (-22.6688, 21.575) centre (-22.6687, 22.575) ccw
  line L42 (-23.6688, 22.575) -> (-23.6687, 34.575)
  arc A47 (-22.6687, 35.575) -> (-23.6687, 34.575) centre (-22.6687, 34.575) ccw
  line L43 (-22.6688, 35.575) -> (-10.6688, 35.575)
  arc A48 (-9.6688, 34.575) -> (-10.6687, 35.575) centre (-10.6688, 34.575) ccw
  line L44 (-44.1, 16.525) -> (-32.1, 16.525)
  arc A49 (-31.1, 15.525) -> (-32.1, 16.525) centre (-32.1, 15.525) ccw
  line L45 (-31.1, 15.525) -> (-31.1, 3.525)
  arc A50 (-32.1, 2.525) -> (-31.1, 3.525) centre (-32.1, 3.525) ccw
  line L46 (-32.1, 2.525) -> (-44.1, 2.525)
  arc A51 (-45.1, 3.525) -> (-44.1, 2.525) centre (-44.1, 3.525) ccw
  line L47 (-45.1, 3.525) -> (-45.1, 15.525)
  arc A52 (-44.1, 16.525) -> (-45.1, 15.525) centre (-44.1, 15.525) ccw
  line L48 (-40.625, 72.675) -> (-40.625, 60.675)
  arc A53 (-41.625, 59.675) -> (-40.625, 60.675) centre (-41.625, 60.675) ccw
  line L49 (-41.625, 59.675) -> (-53.625, 59.675)
  arc A54 (-54.625, 60.675) -> (-53.625, 59.675) centre (-53.625, 60.675) ccw
  line L50 (-54.625, 60.675) -> (-54.625, 72.675)
  arc A55 (-53.625, 73.675) -> (-54.625, 72.675) centre (-53.625, 72.675) ccw
  line L51 (-53.625, 73.675) -> (-41.625, 73.675)
  arc A56 (-40.625, 72.675) -> (-41.625, 73.675) centre (-41.625, 72.675) ccw
  line L52 (-54.9125, 34.575) -> (-54.9125, 22.575)
  arc A57 (-55.9125, 21.575) -> (-54.9125, 22.575) centre (-55.9125, 22.575) ccw
  line L53 (-55.9125, 21.575) -> (-67.9125, 21.575)
  arc A58 (-68.9125, 22.575) -> (-67.9125, 21.575) centre (-67.9125, 22.575) ccw
  line L54 (-68.9125, 22.575) -> (-68.9125, 34.575)
  arc A59 (-67.9125, 35.575) -> (-68.9125, 34.575) centre (-67.9125, 34.575) ccw
  line L55 (-67.9125, 35.575) -> (-55.9125, 35.575)
  arc A60 (-54.9125, 34.575) -> (-55.9125, 35.575) centre (-55.9125, 34.575) ccw
  line L56 (-66.8188, 72.675) -> (-66.8188, 60.675)
  arc A61 (-67.8188, 59.675) -> (-66.8188, 60.675) centre (-67.8188, 60.675) ccw
  line L57 (-67.8188, 59.675) -> (-79.8188, 59.675)
  arc A62 (-80.8188, 60.675) -> (-79.8188, 59.675) centre (-79.8188, 60.675) ccw
  line L58 (-80.8187, 60.675) -> (-80.8187, 72.675)
  arc A63 (-79.8188, 73.675) -> (-80.8188, 72.675) centre (-79.8188, 72.675) ccw
  line L59 (-79.8188, 73.675) -> (-67.8188, 73.675)
  arc A64 (-66.8188, 72.675) -> (-67.8188, 73.675) centre (-67.8188, 72.675) ccw
  line L60 (-88.25, 15.525) -> (-88.25, 3.525)
  arc A65 (-89.25, 2.525) -> (-88.25, 3.525) centre (-89.25, 3.525) ccw
  line L61 (-89.25, 2.525) -> (-101.25, 2.525)
  arc A66 (-102.25, 3.525) -> (-101.25, 2.525) centre (-101.25, 3.525) ccw
  line L62 (-102.25, 3.525) -> (-102.25, 15.525)
  arc A67 (-101.25, 16.525) -> (-102.25, 15.525) centre (-101.25, 15.525) ccw
  line L63 (-101.25, 16.525) -> (-89.25, 16.525)
  arc A68 (-88.25, 15.525) -> (-89.25, 16.525) centre (-89.25, 15.525) ccw
  line L64 (-121.5875, 53.625) -> (-121.5875, 41.625)
  arc A69 (-122.5875, 40.625) -> (-121.5875, 41.625) centre (-122.5875, 41.625) ccw
  line L65 (-122.5875, 40.625) -> (-134.5875, 40.625)
  arc A70 (-135.5875, 41.625) -> (-134.5875, 40.625) centre (-134.5875, 41.625) ccw
  line L66 (-135.5875, 41.625) -> (-135.5875, 53.625)
  arc A71 (-134.5875, 54.625) -> (-135.5875, 53.625) centre (-134.5875, 53.625) ccw
  line L67 (-134.5875, 54.625) -> (-122.5875, 54.625)
  arc A72 (-121.5875, 53.625) -> (-122.5875, 54.625) centre (-122.5875, 53.625) ccw
  line L68 (-150.1625, 34.575) -> (-150.1625, 22.575)
  arc A73 (-151.1625, 21.575) -> (-150.1625, 22.575) centre (-151.1625, 22.575) ccw
  line L69 (-151.1625, 21.575) -> (-163.1625, 21.575)
  arc A74 (-164.1625, 22.575) -> (-163.1625, 21.575) centre (-163.1625, 22.575) ccw
  line L70 (-164.1625, 22.575) -> (-164.1625, 34.575)
  arc A75 (-163.1625, 35.575) -> (-164.1625, 34.575) centre (-163.1625, 34.575) ccw
  line L71 (-163.1625, 35.575) -> (-151.1625, 35.575)
  arc A76 (-150.1625, 34.575) -> (-151.1625, 35.575) centre (-151.1625, 34.575) ccw
  line L72 (-171.5938, 72.675) -> (-171.5937, 60.675)
  arc A77 (-172.5937, 59.675) -> (-171.5937, 60.675) centre (-172.5937, 60.675) ccw
  line L73 (-172.5938, 59.675) -> (-184.5938, 59.675)
  arc A78 (-185.5938, 60.675) -> (-184.5938, 59.675) centre (-184.5938, 60.675) ccw
  line L74 (-185.5938, 60.675) -> (-185.5937, 72.675)
  arc A79 (-184.5938, 73.675) -> (-185.5937, 72.675) centre (-184.5937, 72.675) ccw
  line L75 (-184.5938, 73.675) -> (-172.5937, 73.675)
  arc A80 (-171.5938, 72.675) -> (-172.5937, 73.675) centre (-172.5937, 72.675) ccw
  line L76 (-183.5, 15.525) -> (-183.5, 3.525)
  arc A81 (-184.5, 2.525) -> (-183.5, 3.525) centre (-184.5, 3.525) ccw
  line L77 (-184.5, 2.525) -> (-196.5, 2.525)
  arc A82 (-197.5, 3.525) -> (-196.5, 2.525) centre (-196.5, 3.525) ccw
  line L78 (-197.5, 3.525) -> (-197.5, 15.525)
  arc A83 (-196.5, 16.525) -> (-197.5, 15.525) centre (-196.5, 15.525) ccw
  line L79 (-196.5, 16.525) -> (-184.5, 16.525)
  arc A84 (-183.5, 15.525) -> (-184.5, 16.525) centre (-184.5, 15.525) ccw
  line L80 (-223.9813, 72.675) -> (-223.9813, 60.675)
  arc A85 (-224.9813, 59.675) -> (-223.9812, 60.675) centre (-224.9812, 60.675) ccw
  line L81 (-224.9813, 59.675) -> (-236.9813, 59.675)
  arc A86 (-237.9813, 60.675) -> (-236.9813, 59.675) centre (-236.9813, 60.675) ccw
  line L82 (-237.9813, 60.675) -> (-237.9812, 72.675)
  arc A87 (-236.9813, 73.675) -> (-237.9813, 72.675) centre (-236.9813, 72.675) ccw
  line L83 (-236.9813, 73.675) -> (-224.9813, 73.675)
  arc A88 (-223.9813, 72.675) -> (-224.9813, 73.675) centre (-224.9812, 72.675) ccw
  line L84 (-226.3625, 15.525) -> (-226.3625, 3.525)
  arc A89 (-227.3625, 2.525) -> (-226.3625, 3.525) centre (-227.3625, 3.525) ccw
  line L85 (-227.3625, 2.525) -> (-239.3625, 2.525)
  arc A90 (-240.3625, 3.525) -> (-239.3625, 2.525) centre (-239.3625, 3.525) ccw
  line L86 (-240.3625, 3.525) -> (-240.3625, 15.525)
  arc A91 (-239.3625, 16.525) -> (-240.3625, 15.525) centre (-239.3625, 15.525) ccw
  line L87 (-239.3625, 16.525) -> (-227.3625, 16.525)
  arc A92 (-226.3625, 15.525) -> (-227.3625, 16.525) centre (-227.3625, 15.525) ccw
  line L88 (-260.3688, 35.575) -> (-230.1688, 35.575)
  arc A93 (-229.1688, 34.575) -> (-230.1688, 35.575) centre (-230.1688, 34.575) ccw
  line L89 (-229.1688, 34.575) -> (-229.1688, 22.575)
  arc A94 (-230.1688, 21.575) -> (-229.1688, 22.575) centre (-230.1688, 22.575) ccw
  line L90 (-230.1688, 21.575) -> (-260.3688, 21.575)
  arc A95 (-261.3688, 22.575) -> (-260.3688, 21.575) centre (-260.3688, 22.575) ccw
  line L91 (-261.3688, 22.575) -> (-261.3688, 34.575)
  arc A96 (-260.3688, 35.575) -> (-261.3688, 34.575) centre (-260.3687, 34.575) ccw
  line L92 (-207.3125, 34.575) -> (-207.3125, 22.575)
  arc A97 (-208.3125, 21.575) -> (-207.3125, 22.575) centre (-208.3125, 22.575) ccw
  line L93 (-208.3125, 21.575) -> (-220.3125, 21.575)
  arc A98 (-221.3125, 22.575) -> (-220.3125, 21.575) centre (-220.3125, 22.575) ccw
  line L94 (-221.3125, 22.575) -> (-221.3125, 34.575)
  arc A99 (-220.3125, 35.575) -> (-221.3125, 34.575) centre (-220.3125, 34.575) ccw
  line L95 (-220.3125, 35.575) -> (-208.3125, 35.575)
  arc A100 (-207.3125, 34.575) -> (-208.3125, 35.575) centre (-208.3125, 34.575) ccw
  line L96 (-197.7875, 53.625) -> (-197.7875, 41.625)
  arc A101 (-198.7875, 40.625) -> (-197.7875, 41.625) centre (-198.7875, 41.625) ccw
  line L97 (-198.7875, 40.625) -> (-210.7875, 40.625)
  arc A102 (-211.7875, 41.625) -> (-210.7875, 40.625) centre (-210.7875, 41.625) ccw
  line L98 (-211.7875, 41.625) -> (-211.7875, 53.625)
  arc A103 (-210.7875, 54.625) -> (-211.7875, 53.625) centre (-210.7875, 53.625) ccw
  line L99 (-210.7875, 54.625) -> (-198.7875, 54.625)
  arc A104 (-197.7875, 53.625) -> (-198.7875, 54.625) centre (-198.7875, 53.625) ccw
  line L100 (-169.2125, 34.575) -> (-169.2125, 22.575)
  arc A105 (-170.2125, 21.575) -> (-169.2125, 22.575) centre (-170.2125, 22.575) ccw
  line L101 (-170.2125, 21.575) -> (-182.2125, 21.575)
  arc A106 (-183.2125, 22.575) -> (-182.2125, 21.575) centre (-182.2125, 22.575) ccw
  line L102 (-183.2125, 22.575) -> (-183.2125, 34.575)
  arc A107 (-182.2125, 35.575) -> (-183.2125, 34.575) centre (-182.2125, 34.575) ccw
  line L103 (-182.2125, 35.575) -> (-170.2125, 35.575)
  arc A108 (-169.2125, 34.575) -> (-170.2125, 35.575) centre (-170.2125, 34.575) ccw
  line L104 (-132.5375, 59.675) -> (-162.7375, 59.675)
  arc A109 (-163.7375, 60.675) -> (-162.7375, 59.675) centre (-162.7375, 60.675) ccw
  line L105 (-163.7375, 60.675) -> (-163.7375, 72.675)
  arc A110 (-162.7375, 73.675) -> (-163.7375, 72.675) centre (-162.7375, 72.675) ccw
  line L106 (-162.7375, 73.675) -> (-132.5375, 73.675)
  arc A111 (-131.5375, 72.675) -> (-132.5375, 73.675) centre (-132.5375, 72.675) ccw
  line L107 (-131.5375, 72.675) -> (-131.5375, 60.675)
  arc A112 (-132.5375, 59.675) -> (-131.5375, 60.675) centre (-132.5375, 60.675) ccw
  line L108 (-126.35, 15.525) -> (-126.35, 3.525)
  arc A113 (-127.35, 2.525) -> (-126.35, 3.525) centre (-127.35, 3.525) ccw
  line L109 (-127.35, 2.525) -> (-139.35, 2.525)
  arc A114 (-140.35, 3.525) -> (-139.35, 2.525) centre (-139.35, 3.525) ccw
  line L110 (-140.35, 3.525) -> (-140.35, 15.525)
  arc A115 (-139.35, 16.525) -> (-140.35, 15.525) centre (-139.35, 15.525) ccw
  line L111 (-139.35, 16.525) -> (-127.35, 16.525)
  arc A116 (-126.35, 15.525) -> (-127.35, 16.525) centre (-127.35, 15.525) ccw
  line L112 (-112.0625, 34.575) -> (-112.0625, 22.575)
  arc A117 (-113.0625, 21.575) -> (-112.0625, 22.575) centre (-113.0625, 22.575) ccw
  line L113 (-113.0625, 21.575) -> (-125.0625, 21.575)
  arc A118 (-126.0625, 22.575) -> (-125.0625, 21.575) centre (-125.0625, 22.575) ccw
  line L114 (-126.0625, 22.575) -> (-126.0625, 34.575)
  arc A119 (-125.0625, 35.575) -> (-126.0625, 34.575) centre (-125.0625, 34.575) ccw
  line L115 (-125.0625, 35.575) -> (-113.0625, 35.575)
  arc A120 (-112.0625, 34.575) -> (-113.0625, 35.575) centre (-113.0625, 34.575) ccw
  line L116 (-83.4875, 53.625) -> (-83.4875, 41.625)
  arc A121 (-84.4875, 40.625) -> (-83.4875, 41.625) centre (-84.4875, 41.625) ccw
  line L117 (-84.4875, 40.625) -> (-96.4875, 40.625)
  arc A122 (-97.4875, 41.625) -> (-96.4875, 40.625) centre (-96.4875, 41.625) ccw
  line L118 (-97.4875, 41.625) -> (-97.4875, 53.625)
  arc A123 (-96.4875, 54.625) -> (-97.4875, 53.625) centre (-96.4875, 53.625) ccw
  line L119 (-96.4875, 54.625) -> (-84.4875, 54.625)
  arc A124 (-83.4875, 53.625) -> (-84.4875, 54.625) centre (-84.4875, 53.625) ccw
  line L120 (-73.9625, 34.575) -> (-73.9625, 22.575)
  arc A125 (-74.9625, 21.575) -> (-73.9625, 22.575) centre (-74.9625, 22.575) ccw
  line L121 (-74.9625, 21.575) -> (-86.9625, 21.575)
  arc A126 (-87.9625, 22.575) -> (-86.9625, 21.575) centre (-86.9625, 22.575) ccw
  line L122 (-87.9625, 22.575) -> (-87.9625, 34.575)
  arc A127 (-86.9625, 35.575) -> (-87.9625, 34.575) centre (-86.9625, 34.575) ccw
  line L123 (-86.9625, 35.575) -> (-74.9625, 35.575)
  arc A128 (-73.9625, 34.575) -> (-74.9625, 35.575) centre (-74.9625, 34.575) ccw
  line L124 (-35.8625, 34.575) -> (-35.8625, 22.575)
  arc A129 (-36.8625, 21.575) -> (-35.8625, 22.575) centre (-36.8625, 22.575) ccw
  line L125 (-36.8625, 21.575) -> (-48.8625, 21.575)
  arc A130 (-49.8625, 22.575) -> (-48.8625, 21.575) centre (-48.8625, 22.575) ccw
  line L126 (-49.8625, 22.575) -> (-49.8625, 34.575)
  arc A131 (-48.8625, 35.575) -> (-49.8625, 34.575) centre (-48.8625, 34.575) ccw
  line L127 (-48.8625, 35.575) -> (-36.8625, 35.575)
  arc A132 (-35.8625, 34.575) -> (-36.8625, 35.575) centre (-36.8625, 34.575) ccw
  line L128 (-6.3312, 40.625) -> (-36.5313, 40.625)
  arc A133 (-37.5313, 41.625) -> (-36.5313, 40.625) centre (-36.5313, 41.625) ccw
  line L129 (-37.5312, 41.625) -> (-37.5312, 53.625)
  arc A134 (-36.5313, 54.625) -> (-37.5313, 53.625) centre (-36.5313, 53.625) ccw
  line L130 (-36.5313, 54.625) -> (-6.3313, 54.625)
  arc A135 (-5.3313, 53.625) -> (-6.3313, 54.625) centre (-6.3312, 53.625) ccw
  line L131 (-5.3313, 53.625) -> (-5.3312, 41.625)
  arc A136 (-6.3312, 40.625) -> (-5.3312, 41.625) centre (-6.3312, 41.625) ccw
  line L132 (-7.2875, 15.525) -> (-7.2875, 3.525)
  arc A137 (-8.2875, 2.525) -> (-7.2875, 3.525) centre (-8.2875, 3.525) ccw
  line L133 (-8.2875, 2.525) -> (-20.2875, 2.525)
  arc A138 (-21.2875, 3.525) -> (-20.2875, 2.525) centre (-20.2875, 3.525) ccw
  line L134 (-21.2875, 3.525) -> (-21.2875, 15.525)
  arc A139 (-20.2875, 16.525) -> (-21.2875, 15.525) centre (-20.2875, 15.525) ccw
  line L135 (-20.2875, 16.525) -> (-8.2875, 16.525)
  arc A140 (-7.2875, 15.525) -> (-8.2875, 16.525) centre (-8.2875, 15.525) ccw
  line L136 (-14.4313, 72.675) -> (-14.4313, 60.675)
  arc A141 (-15.4313, 59.675) -> (-14.4313, 60.675) centre (-15.4312, 60.675) ccw
  line L137 (-15.4313, 59.675) -> (-27.4313, 59.675)
  arc A142 (-28.4313, 60.675) -> (-27.4313, 59.675) centre (-27.4313, 60.675) ccw
  line L138 (-28.4313, 60.675) -> (-28.4312, 72.675)
  arc A143 (-27.4313, 73.675) -> (-28.4312, 72.675) centre (-27.4312, 72.675) ccw
  line L139 (-27.4313, 73.675) -> (-15.4313, 73.675)
  arc A144 (-14.4313, 72.675) -> (-15.4313, 73.675) centre (-15.4313, 72.675) ccw
  line L140 (-50.15, 15.525) -> (-50.15, 3.525)
  arc A145 (-51.15, 2.525) -> (-50.15, 3.525) centre (-51.15, 3.525) ccw
  line L141 (-51.15, 2.525) -> (-63.15, 2.525)
  arc A146 (-64.15, 3.525) -> (-63.15, 2.525) centre (-63.15, 3.525) ccw
  line L142 (-64.15, 3.525) -> (-64.15, 15.525)
  arc A147 (-63.15, 16.525) -> (-64.15, 15.525) centre (-63.15, 15.525) ccw
  line L143 (-63.15, 16.525) -> (-51.15, 16.525)
  arc A148 (-50.15, 15.525) -> (-51.15, 16.525) centre (-51.15, 15.525) ccw
  line L144 (-64.4375, 53.625) -> (-64.4375, 41.625)
  arc A149 (-65.4375, 40.625) -> (-64.4375, 41.625) centre (-65.4375, 41.625) ccw
  line L145 (-65.4375, 40.625) -> (-77.4375, 40.625)
  arc A150 (-78.4375, 41.625) -> (-77.4375, 40.625) centre (-77.4375, 41.625) ccw
  line L146 (-78.4375, 41.625) -> (-78.4375, 53.625)
  arc A151 (-77.4375, 54.625) -> (-78.4375, 53.625) centre (-77.4375, 53.625) ccw
  line L147 (-77.4375, 54.625) -> (-65.4375, 54.625)
  arc A152 (-64.4375, 53.625) -> (-65.4375, 54.625) centre (-65.4375, 53.625) ccw
  line L148 (-93.0125, 34.575) -> (-93.0125, 22.575)
  arc A153 (-94.0125, 21.575) -> (-93.0125, 22.575) centre (-94.0125, 22.575) ccw
  line L149 (-94.0125, 21.575) -> (-106.0125, 21.575)
  arc A154 (-107.0125, 22.575) -> (-106.0125, 21.575) centre (-106.0125, 22.575) ccw
  line L150 (-107.0125, 22.575) -> (-107.0125, 34.575)
  arc A155 (-106.0125, 35.575) -> (-107.0125, 34.575) centre (-106.0125, 34.575) ccw
  line L151 (-106.0125, 35.575) -> (-94.0125, 35.575)
  arc A156 (-93.0125, 34.575) -> (-94.0125, 35.575) centre (-94.0125, 34.575) ccw
  line L152 (-102.5375, 53.625) -> (-102.5375, 41.625)
  arc A157 (-103.5375, 40.625) -> (-102.5375, 41.625) centre (-103.5375, 41.625) ccw
  line L153 (-103.5375, 40.625) -> (-115.5375, 40.625)
  arc A158 (-116.5375, 41.625) -> (-115.5375, 40.625) centre (-115.5375, 41.625) ccw
  line L154 (-116.5375, 41.625) -> (-116.5375, 53.625)
  arc A159 (-115.5375, 54.625) -> (-116.5375, 53.625) centre (-115.5375, 53.625) ccw
  line L155 (-115.5375, 54.625) -> (-103.5375, 54.625)
  arc A160 (-102.5375, 53.625) -> (-103.5375, 54.625) centre (-103.5375, 53.625) ccw
  line L156 (-145.4, 15.525) -> (-145.4, 3.525)
  arc A161 (-146.4, 2.525) -> (-145.4, 3.525) centre (-146.4, 3.525) ccw
  line L157 (-146.4, 2.525) -> (-158.4, 2.525)
  arc A162 (-159.4, 3.525) -> (-158.4, 2.525) centre (-158.4, 3.525) ccw
  line L158 (-159.4, 3.525) -> (-159.4, 15.525)
  arc A163 (-158.4, 16.525) -> (-159.4, 15.525) centre (-158.4, 15.525) ccw
  line L159 (-158.4, 16.525) -> (-146.4, 16.525)
  arc A164 (-145.4, 15.525) -> (-146.4, 16.525) centre (-146.4, 15.525) ccw
  line L160 (-159.6875, 53.625) -> (-159.6875, 41.625)
  arc A165 (-160.6875, 40.625) -> (-159.6875, 41.625) centre (-160.6875, 41.625) ccw
  line L161 (-160.6875, 40.625) -> (-172.6875, 40.625)
  arc A166 (-173.6875, 41.625) -> (-172.6875, 40.625) centre (-172.6875, 41.625) ccw
  line L162 (-173.6875, 41.625) -> (-173.6875, 53.625)
  arc A167 (-172.6875, 54.625) -> (-173.6875, 53.625) centre (-172.6875, 53.625) ccw
  line L163 (-172.6875, 54.625) -> (-160.6875, 54.625)
  arc A168 (-159.6875, 53.625) -> (-160.6875, 54.625) centre (-160.6875, 53.625) ccw
  line L164 (-164.45, 15.525) -> (-164.45, 3.525)
  arc A169 (-165.45, 2.525) -> (-164.45, 3.525) centre (-165.45, 3.525) ccw
  line L165 (-165.45, 2.525) -> (-177.45, 2.525)
  arc A170 (-178.45, 3.525) -> (-177.45, 2.525) centre (-177.45, 3.525) ccw
  line L166 (-178.45, 3.525) -> (-178.45, 15.525)
  arc A171 (-177.45, 16.525) -> (-178.45, 15.525) centre (-177.45, 15.525) ccw
  line L167 (-177.45, 16.525) -> (-165.45, 16.525)
  arc A172 (-164.45, 15.525) -> (-165.45, 16.525) centre (-165.45, 15.525) ccw
  line L168 (-197.7875, 72.675) -> (-197.7875, 60.675)
  arc A173 (-198.7875, 59.675) -> (-197.7875, 60.675) centre (-198.7875, 60.675) ccw
  line L169 (-198.7875, 59.675) -> (-210.7875, 59.675)
  arc A174 (-211.7875, 60.675) -> (-210.7875, 59.675) centre (-210.7875, 60.675) ccw
  line L170 (-211.7875, 60.675) -> (-211.7875, 72.675)
  arc A175 (-210.7875, 73.675) -> (-211.7875, 72.675) centre (-210.7875, 72.675) ccw
  line L171 (-210.7875, 73.675) -> (-198.7875, 73.675)
  arc A176 (-197.7875, 72.675) -> (-198.7875, 73.675) centre (-198.7875, 72.675) ccw
  line L172 (-202.55, 15.525) -> (-202.55, 3.525)
  arc A177 (-203.55, 2.525) -> (-202.55, 3.525) centre (-203.55, 3.525) ccw
  line L173 (-203.55, 2.525) -> (-215.55, 2.525)